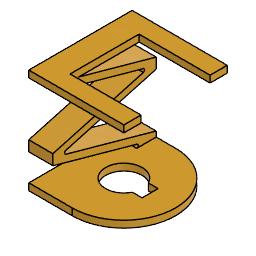
Keybord-Base (Autodesk Fusion 360 archive; units mm, degrees)
design "ボタン-スプリング"
Autodesk Fusion 360 part; units mm, degrees
note: some values were not read from the file. Set by a fixed rule: which face or edge a step refers to.
(part 1 of 3)
sketch "スケッチ1" plane through (0, 0, 0) normal (0, 0, 1) x (1, 0, 0)
  circle A0 centre (0, 0) radius 2.65
  line L0 (0, -7.5) -> (0, 7.5)
  line L1 (0, 7.5) -> (-6.3, 7.5)
  line L2 (-6.3, 7.5) -> (-6.3, -7.5)
  line L3 (-6.3, -7.5) -> (0, -7.5)
  line L4 (0, -7.5) -> (0, 7.5)
  arc A1 (0, -7.5) -> (0, 7.5) centre (0, 0) ccw
  line L5 (2.65, 0) -> (-2.65, 0)
  line L6 (3.8, 1.15) -> (1.5, 1.15)
  line L7 (1.5, 1.15) -> (1.5, -1.15)
  line L8 (1.5, -1.15) -> (3.8, -1.15)
  line L9 (3.8, -1.15) -> (3.8, 1.15)
  line L10 (3.8, 1.15) -> (1.5, -1.15) construction
  line L11 (1.5, 1.15) -> (3.8, -1.15) construction
  point P0 (2.65, 0)
  dimension "d1" = 5.3
  dimension "d2" = 15
  dimension "d5" = 6.3
  dimension "d6" = 15
  dimension "d31" = 2.3
  dimension "d32" = 2.3
  constraint coincident A0.centre A1.centre
  constraint midpoint L0 A0.centre
  constraint vertical L0
  constraint horizontal L1
  constraint vertical L2
  constraint horizontal L3
  constraint vertical L4
  constraint midpoint L5 A0.centre
  constraint coincident A0 L5.end
  constraint perpendicular L0 L5
  constraint horizontal L6
  constraint perpendicular L6 L7
  constraint parallel L6 L8
  constraint parallel L7 L9
  constraint coincident L10 P0
  constraint coincident L11 P0
  constraint coincident P0 L5.start
  measures "d1" diameter of A0
  measures "d2" diameter of A1
  measures "d5" distance of A0.centre L2
  measures "d6" distance of L1 L3
  measures "d31" distance of L7.end L8.end
  measures "d32" distance of L6.end L7.end
extrude "押し出し1" add sketch "スケッチ1" along normal blind 1 contours A0 L0 L4 A1 L6 L8 L9 | A0 L0 L1 L2 L3 L4
sketch "スケッチ2" plane through (-6.3, 0, 0) normal (-1, 0, 0) x (0, -1, 0)
  line L0 (-7.5, 0) -> (7.5, 0)
  line L1 (7.5, 0) -> (7.5, 1)
  line L2 (7.5, 1) -> (-7.5, 1)
  line L3 (-7.5, 1) -> (-7.5, 0)
  line L4 (-7.5, 1) -> (-7.5, 16) construction
  line L5 (7.5, 1) -> (7.5, 16) construction
  line L6 (-7.5, 1) -> (-7.5, 1.7604)
  line L7 (-6.5, 1) -> (-7.5, 1)
  line L8 (-7.5, 1) -> (-7.5, 1.7604)
  line L9 (-4.7298, 1.4909) -> (7.5, 4.8825)
  line L10 (-4.663, 1) -> (10.2045, 1) construction
  line L11 (-7.5, 1.7604) -> (5.6313, 5.4021)
  line L12 (5.6313, 5.8839) -> (-7.5, 9.5255)
  line L13 (-5.6313, 10.045) -> (7.5, 6.4034)
  line L14 (7.5, 6.4034) -> (7.5, 4.8825)
  line L15 (-5.6313, 10.5268) -> (7.5, 14.1685)
  line L16 (-7.5, 11.0463) -> (3.758, 14.1685)
  line L17 (-7.5, 11.0463) -> (-7.5, 9.5255)
  line L18 (7.5, 14.1685) -> (3.758, 14.1685)
  arc A0 (-4.7298, 1.4909) -> (-4.663, 1) centre (-4.663, 1.25) ccw
  arc A1 (5.6313, 5.4021) -> (5.6313, 5.8839) centre (5.5645, 5.643) ccw
  arc A2 (-5.6313, 10.5268) -> (-5.6313, 10.045) centre (-5.5645, 10.2859) ccw
  point P0 (6.5, 5.643)
  point P1 (-6.5, 10.2859)
  dimension "d7" = 15
  dimension "d8" = 15
  dimension "d9" = 15.5
  dimension "d15" = 15.5
  dimension "d16" = 1
  dimension "d17" = 1
  dimension "d18" = 15.5
  dimension "d19" = 15.5
  dimension "d20" = 1
  dimension "d21" = 1
  dimension "d22" = 15.5
  dimension "d23" = 15.5
  dimension "d24" = 1
  dimension "d25" = 1
  dimension "d26" = 0.25
  dimension "d27" = 0.25
  dimension "d28" = 0.25
  constraint coincident L2.end L3.start
  constraint perpendicular L2 L4
  constraint coincident L1.end L2.start
  constraint perpendicular L2 L5
  constraint coincident L4 L6.end
  constraint horizontal L7
  constraint vertical L8
  constraint coincident L2 L7.start
  constraint horizontal L10
  constraint coincident L5 L9.end
  constraint coincident L5 L13.end
  constraint coincident L4 L12.end
  constraint coincident L4 L16.start
  constraint coincident L5 L15.end
  constraint parallel L10 L18
  constraint coincident L7.start L9
  constraint coincident L7.start L10
  constraint tangent L9 A0
  constraint tangent L10 A0
  constraint coincident P0 L11
  constraint coincident P0 L12
  constraint tangent L11 A1
  constraint tangent L12 A1
  constraint coincident P1 L15
  constraint coincident P1 L13
  constraint tangent L15 A2
  constraint tangent L13 A2
  measures "d7" distance of L2.end L4.end
  measures "d8" distance of L1.end L5.end
  measures "d9" angle of L9 L10
  measures "d15" angle of L10 L11
  measures "d16" distance of L9 L11
  measures "d17" distance of L7.start L2.end
  measures "d18" angle of L10 L12
  measures "d19" angle of L10 L13
  measures "d20" distance of L12 L13
  measures "d21" distance of P0 L14
  measures "d22" angle of L10 L15
  measures "d23" angle of L10 L16
  measures "d24" distance of L15 L16
  measures "d25" distance of P1 L17
  measures "d26" radius of A0
  measures "d27" radius of A1
  measures "d28" radius of A2
extrude "押し出し2" add sketch "スケッチ2" against normal blind 3.5 contours L2 L6 L7 L8 L9 L11 L12 L13 L14 L15 L16 L17 L18 A0 A1 A2
sketch "スケッチ3" plane through (0, 0, 14.1685) normal (0, 0, 1) x (-1, 0, 0)
  line L0 (6.3, 3.758) -> (6.3, 7.5)
  line L1 (6.3, 7.5) -> (2.8, 7.5)
  line L2 (2.8, 7.5) -> (2.8, 3.758)
  line L3 (2.8, 3.758) -> (6.3, 3.758)
  line L4 (2.8, -4.663) -> (6.3, -4.663)
  line L5 (6.3, -4.663) -> (6.3, 7.5)
  line L6 (6.3, 7.5) -> (0, 7.5)
  arc A0 (0, 7.5) -> (0, -7.5) centre (0, 0) ccw
  line L7 (0, -7.5) -> (2.8, -7.5)
  line L8 (2.8, -7.5) -> (2.8, -4.663)
  line L9 (-3.8, -1.15) -> (-3.8, 1.15)
  line L10 (-3.8, 1.15) -> (-2.3875, 1.15)
  arc A1 (-2.3875, -1.15) -> (-2.3875, 1.15) centre (0, 0) ccw
  line L11 (-2.3875, -1.15) -> (-3.8, -1.15)
  line L12 (6.3, -7.5) -> (6.3, 3.758)
  line L13 (6.3, 3.758) -> (2.8, 3.758)
  line L14 (2.8, 3.758) -> (2.8, -7.5)
  line L15 (2.8, -7.5) -> (6.3, -7.5)
  line L16 (6.3, 5) -> (6.3, -5)
  line L17 (-7.5, 0) -> (-7.5, -7.5)
  line L18 (-7.5, -7.5) -> (6.3, -7.5)
  line L19 (6.3, -4.663) -> (6.3, -7.5)
  line L20 (6.3, -5) -> (-7.5, -5)
  line L21 (-20, 0) -> (-2.5, 0)
  line L22 (6.3, 5) -> (-7.5, 5)
  line L23 (-7.5, 0) -> (-7.5, 7.5)
  line L24 (6.3, 4.663) -> (6.3, 7.5)
  line L25 (-7.5, 7.5) -> (6.3, 7.5)
  point P0 (6.3, 0)
  dimension "d38" = 5
  constraint midpoint L16 P0
  constraint coincident L12 P0
  constraint coincident L12 L16.end
  constraint midpoint A0 L17.start
  constraint tangent A0 L17
  constraint perpendicular L7 L17
  constraint coincident L12.start L15.end
  constraint perpendicular L12 L18
  constraint coincident L4.end L5.start
  constraint coincident L17 L20.end
  constraint perpendicular L17 L20
  constraint symmetric L17.start L21 L23.start
  constraint symmetric L17.end L21 L23.end
  constraint symmetric L12.start L21 L0.end
  constraint symmetric L4.end L21 L24.start
  constraint symmetric L16.end L21 L16.start
  constraint symmetric L20.end L21 L22.end
  measures "d38" distance of A0.centre L20
extrude "押し出し3" add sketch "スケッチ3" along normal blind 1 contours L0 L2 L3 L5 L13 L16 L22 L24 | L3 L4 L5 L12 L13 L14 L16 | L4 L8 L12 L14 L16 L19 L20 | L0 L1 L2 L5 L6 L22 L24 L25 | L2 L6 A0 L22 L25 | L8 L12 L14 L15 L18 L19 L20 | A0 L22 L23 L25 | A0 L7 L8 L14 L18 L20 | A0 L17 L18 L20
equation "d5 = d1 + 1 mm"
equation "d6 = d2"
equation "d8 = d7"
equation "d15 = d9"
equation "d17 = d16"
equation "d18 = d9"
equation "d19 = d9"
equation "d20 = d16"
equation "d21 = d16"
equation "d22 = d9"
equation "d23 = d9"
equation "d24 = d16"
equation "d25 = d16"
equation "d31 = d32"

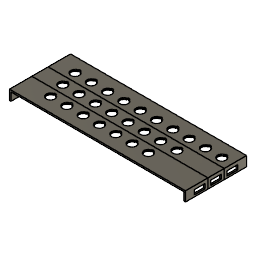
design "Keybord-Base-top"
Autodesk Fusion 360 part; units mm, degrees
sketch "スケッチ1" plane through (0, 0, 0) normal (0, 0, 1) x (1, 0, 0)
  circle A0 centre (0, 0) radius 4.75
  line L0 (1.25, 3.5) -> (-1.25, 3.5)
  line L1 (-1.25, 3.5) -> (-1.25, 6)
  line L2 (-1.25, 6) -> (1.25, 6)
  line L3 (1.25, 6) -> (1.25, 3.5)
  line L4 (1.25, 3.5) -> (-1.25, 6) construction
  line L5 (-1.25, 3.5) -> (1.25, 6) construction
  line L6 (0, -6.2565) -> (0, 6.2565)
  line L7 (-5.8047, 0) -> (5.8047, 0)
  circle A1 centre (20, 0) radius 4.75
  line L8 (18.75, 3.5) -> (21.25, 6) construction
  line L9 (14.1953, 0) -> (25.8047, 0)
  line L10 (20, -6.2565) -> (20, 6.2565)
  line L11 (18.75, 6) -> (21.25, 6)
  line L12 (18.75, 3.5) -> (18.75, 6)
  line L13 (21.25, 3.5) -> (18.75, 6) construction
  line L14 (21.25, 6) -> (21.25, 3.5)
  line L15 (21.25, 3.5) -> (18.75, 3.5)
  circle A2 centre (40, 0) radius 4.75
  line L16 (38.75, 3.5) -> (41.25, 6) construction
  line L17 (34.1953, 0) -> (45.8047, 0)
  line L18 (40, -6.2565) -> (40, 6.2565)
  line L19 (38.75, 6) -> (41.25, 6)
  line L20 (38.75, 3.5) -> (38.75, 6)
  line L21 (41.25, 3.5) -> (38.75, 6) construction
  line L22 (41.25, 6) -> (41.25, 3.5)
  line L23 (41.25, 3.5) -> (38.75, 3.5)
  circle A3 centre (60, 0) radius 4.75
  line L24 (58.75, 3.5) -> (61.25, 6) construction
  line L25 (54.1953, 0) -> (65.8047, 0)
  line L26 (60, -6.2565) -> (60, 6.2565)
  line L27 (58.75, 6) -> (61.25, 6)
  line L28 (58.75, 3.5) -> (58.75, 6)
  line L29 (61.25, 3.5) -> (58.75, 6) construction
  line L30 (61.25, 6) -> (61.25, 3.5)
  line L31 (61.25, 3.5) -> (58.75, 3.5)
  line L32 (-21.25, 3.5) -> (-18.75, 6) construction
  line L33 (-18.75, 6) -> (-18.75, 3.5)
  line L34 (-25.8047, 0) -> (-14.1953, 0)
  line L35 (-21.25, 3.5) -> (-21.25, 6)
  line L36 (-20, -6.2565) -> (-20, 6.2565)
  line L37 (-21.25, 6) -> (-18.75, 6)
  circle A4 centre (-20, 0) radius 4.75
  line L38 (-18.75, 3.5) -> (-21.25, 6) construction
  line L39 (-18.75, 3.5) -> (-21.25, 3.5)
  line L40 (-41.25, 3.5) -> (-38.75, 6) construction
  line L41 (-38.75, 6) -> (-38.75, 3.5)
  line L42 (-45.8047, 0) -> (-34.1953, 0)
  line L43 (-41.25, 3.5) -> (-41.25, 6)
  line L44 (-40, -6.2565) -> (-40, 6.2565)
  line L45 (-41.25, 6) -> (-38.75, 6)
  circle A5 centre (-40, 0) radius 4.75
  line L46 (-38.75, 3.5) -> (-41.25, 6) construction
  line L47 (-38.75, 3.5) -> (-41.25, 3.5)
  line L48 (-61.25, 3.5) -> (-58.75, 6) construction
  line L49 (-58.75, 6) -> (-58.75, 3.5)
  line L50 (-65.8047, 0) -> (-54.1953, 0)
  line L51 (-61.25, 3.5) -> (-61.25, 6)
  line L52 (-60, -6.2565) -> (-60, 6.2565)
  line L53 (-61.25, 6) -> (-58.75, 6)
  circle A6 centre (-60, 0) radius 4.75
  line L54 (-58.75, 3.5) -> (-61.25, 6) construction
  line L55 (-58.75, 3.5) -> (-61.25, 3.5)
  line L56 (-81.25, 3.5) -> (-78.75, 6) construction
  line L57 (-78.75, 6) -> (-78.75, 3.5)
  line L58 (-85.8047, 0) -> (-74.1953, 0)
  line L59 (-81.25, 3.5) -> (-81.25, 6)
  line L60 (-80, -6.2565) -> (-80, 6.2565)
  line L61 (-81.25, 6) -> (-78.75, 6)
  circle A7 centre (-80, 0) radius 4.75
  line L62 (-78.75, 3.5) -> (-81.25, 6) construction
  line L63 (-78.75, 3.5) -> (-81.25, 3.5)
  line L64 (-3.75, 23.5) -> (-6.25, 23.5)
  line L65 (-3.75, 23.5) -> (-6.25, 26) construction
  line L66 (-10.8047, 20) -> (0.8047, 20)
  line L67 (-6.25, 23.5) -> (-6.25, 26)
  line L68 (-6.25, 23.5) -> (-3.75, 26) construction
  line L69 (-6.25, 26) -> (-3.75, 26)
  line L70 (-5, 13.7435) -> (-5, 26.2565)
  line L71 (-3.75, 26) -> (-3.75, 23.5)
  circle A8 centre (-5, 20) radius 4.75
  line L72 (16.25, 23.5) -> (13.75, 23.5)
  line L73 (13.75, 23.5) -> (13.75, 26)
  line L74 (16.25, 23.5) -> (13.75, 26) construction
  circle A9 centre (15, 20) radius 4.75
  line L75 (13.75, 23.5) -> (16.25, 26) construction
  line L76 (9.1953, 20) -> (20.8047, 20)
  line L77 (15, 13.7435) -> (15, 26.2565)
  line L78 (13.75, 26) -> (16.25, 26)
  line L79 (16.25, 26) -> (16.25, 23.5)
  line L80 (36.25, 23.5) -> (33.75, 23.5)
  line L81 (33.75, 23.5) -> (33.75, 26)
  line L82 (36.25, 23.5) -> (33.75, 26) construction
  circle A10 centre (35, 20) radius 4.75
  line L83 (33.75, 23.5) -> (36.25, 26) construction
  line L84 (29.1953, 20) -> (40.8047, 20)
  line L85 (35, 13.7435) -> (35, 26.2565)
  line L86 (33.75, 26) -> (36.25, 26)
  line L87 (36.25, 26) -> (36.25, 23.5)
  line L88 (56.25, 23.5) -> (53.75, 23.5)
  line L89 (53.75, 23.5) -> (53.75, 26)
  line L90 (56.25, 23.5) -> (53.75, 26) construction
  circle A11 centre (55, 20) radius 4.75
  line L91 (53.75, 23.5) -> (56.25, 26) construction
  line L92 (49.1953, 20) -> (60.8047, 20)
  line L93 (55, 13.7435) -> (55, 26.2565)
  line L94 (53.75, 26) -> (56.25, 26)
  line L95 (56.25, 26) -> (56.25, 23.5)
  line L96 (76.25, 23.5) -> (73.75, 23.5)
  line L97 (73.75, 23.5) -> (73.75, 26)
  line L98 (76.25, 23.5) -> (73.75, 26) construction
  circle A12 centre (75, 20) radius 4.75
  line L99 (73.75, 23.5) -> (76.25, 26) construction
  line L100 (69.1953, 20) -> (80.8047, 20)
  line L101 (75, 13.7435) -> (75, 26.2565)
  line L102 (73.75, 26) -> (76.25, 26)
  line L103 (76.25, 26) -> (76.25, 23.5)
  line L104 (96.25, 23.5) -> (93.75, 23.5)
  line L105 (93.75, 23.5) -> (93.75, 26)
  line L106 (96.25, 23.5) -> (93.75, 26) construction
  circle A13 centre (95, 20) radius 4.75
  line L107 (93.75, 23.5) -> (96.25, 26) construction
  line L108 (89.1953, 20) -> (100.8047, 20)
  line L109 (95, 13.7435) -> (95, 26.2565)
  line L110 (93.75, 26) -> (96.25, 26)
  line L111 (96.25, 26) -> (96.25, 23.5)
  line L112 (-23.75, 26) -> (-23.75, 23.5)
  line L113 (-23.75, 23.5) -> (-26.25, 23.5)
  circle A14 centre (-25, 20) radius 4.75
  line L114 (-23.75, 23.5) -> (-26.25, 26) construction
  line L115 (-30.8047, 20) -> (-19.1953, 20)
  line L116 (-25, 13.7435) -> (-25, 26.2565)
  line L117 (-26.25, 23.5) -> (-26.25, 26)
  line L118 (-26.25, 26) -> (-23.75, 26)
  line L119 (-26.25, 23.5) -> (-23.75, 26) construction
  line L120 (-43.75, 26) -> (-43.75, 23.5)
  line L121 (-43.75, 23.5) -> (-46.25, 23.5)
  circle A15 centre (-45, 20) radius 4.75
  line L122 (-43.75, 23.5) -> (-46.25, 26) construction
  line L123 (-50.8047, 20) -> (-39.1953, 20)
  line L124 (-45, 13.7435) -> (-45, 26.2565)
  line L125 (-46.25, 23.5) -> (-46.25, 26)
  line L126 (-46.25, 26) -> (-43.75, 26)
  line L127 (-46.25, 23.5) -> (-43.75, 26) construction
  line L128 (-63.75, 26) -> (-63.75, 23.5)
  line L129 (-63.75, 23.5) -> (-66.25, 23.5)
  circle A16 centre (-65, 20) radius 4.75
  line L130 (-63.75, 23.5) -> (-66.25, 26) construction
  line L131 (-70.8047, 20) -> (-59.1953, 20)
  line L132 (-65, 13.7435) -> (-65, 26.2565)
  line L133 (-66.25, 23.5) -> (-66.25, 26)
  line L134 (-66.25, 26) -> (-63.75, 26)
  line L135 (-66.25, 23.5) -> (-63.75, 26) construction
  line L136 (-83.75, 26) -> (-83.75, 23.5)
  line L137 (-83.75, 23.5) -> (-86.25, 23.5)
  circle A17 centre (-85, 20) radius 4.75
  line L138 (-83.75, 23.5) -> (-86.25, 26) construction
  line L139 (-90.8047, 20) -> (-79.1953, 20)
  line L140 (-85, 13.7435) -> (-85, 26.2565)
  line L141 (-86.25, 23.5) -> (-86.25, 26)
  line L142 (-86.25, 26) -> (-83.75, 26)
  line L143 (-86.25, 23.5) -> (-83.75, 26) construction
  circle A18 centre (5, -20) radius 4.75
  line L144 (3.75, -14) -> (6.25, -14)
  line L145 (6.25, -14) -> (6.25, -16.5)
  line L146 (3.75, -16.5) -> (3.75, -14)
  line L147 (6.25, -16.5) -> (3.75, -16.5)
  line L148 (6.25, -16.5) -> (3.75, -14) construction
  line L149 (3.75, -16.5) -> (6.25, -14) construction
  line L150 (-0.8294, -20) -> (10.7799, -20)
  line L151 (5, -26.3014) -> (5, -13.7884)
  line L152 (26.25, -16.5) -> (23.75, -16.5)
  circle A19 centre (25, -20) radius 4.75
  line L153 (23.75, -14) -> (26.25, -14)
  line L154 (26.25, -16.5) -> (23.75, -14) construction
  line L155 (25, -26.3014) -> (25, -13.7884)
  line L156 (23.75, -16.5) -> (23.75, -14)
  line L157 (23.75, -16.5) -> (26.25, -14) construction
  line L158 (19.1706, -20) -> (30.7799, -20)
  line L159 (26.25, -14) -> (26.25, -16.5)
  line L160 (46.25, -16.5) -> (43.75, -16.5)
  circle A20 centre (45, -20) radius 4.75
  line L161 (43.75, -14) -> (46.25, -14)
  line L162 (46.25, -16.5) -> (43.75, -14) construction
  line L163 (45, -26.3014) -> (45, -13.7884)
  line L164 (43.75, -16.5) -> (43.75, -14)
  line L165 (43.75, -16.5) -> (46.25, -14) construction
  line L166 (39.1706, -20) -> (50.7799, -20)
  line L167 (46.25, -14) -> (46.25, -16.5)
  line L168 (-16.25, -16.5) -> (-16.25, -14)
  line L169 (-13.75, -16.5) -> (-16.25, -14) construction
  circle A21 centre (-15, -20) radius 4.75
  line L170 (-16.25, -16.5) -> (-13.75, -14) construction
  line L171 (-15, -26.3014) -> (-15, -13.7884)
  line L172 (-16.25, -14) -> (-13.75, -14)
  line L173 (-13.75, -16.5) -> (-16.25, -16.5)
  line L174 (-13.75, -14) -> (-13.75, -16.5)
  line L175 (-20.8294, -20) -> (-9.2201, -20)
  line L176 (-36.25, -16.5) -> (-36.25, -14)
  line L177 (-33.75, -16.5) -> (-36.25, -14) construction
  circle A22 centre (-35, -20) radius 4.75
  line L178 (-36.25, -16.5) -> (-33.75, -14) construction
  line L179 (-35, -26.3014) -> (-35, -13.7884)
  line L180 (-36.25, -14) -> (-33.75, -14)
  line L181 (-33.75, -16.5) -> (-36.25, -16.5)
  line L182 (-33.75, -14) -> (-33.75, -16.5)
  line L183 (-40.8294, -20) -> (-29.2201, -20)
  line L184 (-56.25, -16.5) -> (-56.25, -14)
  line L185 (-53.75, -16.5) -> (-56.25, -14) construction
  circle A23 centre (-55, -20) radius 4.75
  line L186 (-56.25, -16.5) -> (-53.75, -14) construction
  line L187 (-55, -26.3014) -> (-55, -13.7884)
  line L188 (-56.25, -14) -> (-53.75, -14)
  line L189 (-53.75, -16.5) -> (-56.25, -16.5)
  line L190 (-53.75, -14) -> (-53.75, -16.5)
  line L191 (-60.8294, -20) -> (-49.2201, -20)
  line L192 (-76.25, -16.5) -> (-76.25, -14)
  line L193 (-73.75, -16.5) -> (-76.25, -14) construction
  circle A24 centre (-75, -20) radius 4.75
  line L194 (-76.25, -16.5) -> (-73.75, -14) construction
  line L195 (-75, -26.3014) -> (-75, -13.7884)
  line L196 (-76.25, -14) -> (-73.75, -14)
  line L197 (-73.75, -16.5) -> (-76.25, -16.5)
  line L198 (-73.75, -14) -> (-73.75, -16.5)
  line L199 (-80.8294, -20) -> (-69.2201, -20)
  line L200 (108, 37.5) -> (-108, 37.5)
  line L201 (-108, 37.5) -> (-108, -37.5)
  line L202 (-108, -37.5) -> (108, -37.5)
  line L203 (108, -37.5) -> (108, 37.5)
  line L204 (108, 37.5) -> (-108, -37.5) construction
  line L205 (-108, 37.5) -> (108, -37.5) construction
  point P0 (0, 4.75)
  point P1 (20, 0)
  point P2 (20, 0)
  point P3 (20, 4.75)
  point P4 (20, 0)
  point P5 (20, 0)
  point P6 (40, 0)
  point P7 (40, 0)
  point P8 (40, 4.75)
  point P9 (40, 0)
  point P10 (40, 0)
  point P11 (60, 0)
  point P12 (60, 0)
  point P13 (60, 4.75)
  point P14 (60, 0)
  point P15 (60, 0)
  point P16 (-20, 0)
  point P17 (-20, 0)
  point P18 (-20, 0)
  point P19 (-20, 0)
  point P20 (-20, 4.75)
  point P21 (-40, 0)
  point P22 (-40, 0)
  point P23 (-40, 0)
  point P24 (-40, 0)
  point P25 (-40, 4.75)
  point P26 (-60, 0)
  point P27 (-60, 0)
  point P28 (-60, 0)
  point P29 (-60, 0)
  point P30 (-60, 4.75)
  point P31 (-80, 0)
  point P32 (-80, 0)
  point P33 (-80, 0)
  point P34 (-80, 0)
  point P35 (-80, 4.75)
  point P36 (25.8047, 17)
  point P37 (-5, 20)
  point P38 (14.1953, 17)
  point P39 (-5, 24.75)
  point P40 (-5, 20)
  point P41 (-5, 20)
  point P42 (-5, 20)
  point P43 (15, 24.75)
  point P44 (15, 20)
  point P45 (15, 20)
  point P46 (15, 20)
  point P47 (15, 20)
  point P48 (35, 24.75)
  point P49 (35, 20)
  point P50 (35, 20)
  point P51 (35, 20)
  point P52 (35, 20)
  point P53 (55, 24.75)
  point P54 (55, 20)
  point P55 (55, 20)
  point P56 (55, 20)
  point P57 (55, 20)
  point P58 (75, 24.75)
  point P59 (75, 20)
  point P60 (75, 20)
  point P61 (75, 20)
  point P62 (75, 20)
  point P63 (95, 24.75)
  point P64 (95, 20)
  point P65 (95, 20)
  point P66 (95, 20)
  point P67 (95, 20)
  point P68 (-25, 20)
  point P69 (-25, 20)
  point P70 (-25, 24.75)
  point P71 (-25, 20)
  point P72 (-25, 20)
  point P73 (-45, 20)
  point P74 (-45, 20)
  point P75 (-45, 24.75)
  point P76 (-45, 20)
  point P77 (-45, 20)
  point P78 (-65, 20)
  point P79 (-65, 20)
  point P80 (-65, 24.75)
  point P81 (-65, 20)
  point P82 (-65, 20)
  point P83 (-85, 20)
  point P84 (-85, 20)
  point P85 (-85, 24.75)
  point P86 (-85, 20)
  point P87 (-85, 20)
  point P88 (5, -15.25)
  point P89 (25, -15.25)
  point P90 (45, -15.25)
  point P91 (-15, -15.25)
  point P92 (-35, -15.25)
  point P93 (-55, -15.25)
  point P94 (-75, -15.25)
  dimension "d1" = 9.5
  dimension "d2" = 2.5
  dimension "d3" = 2.5
  dimension "d10" = 20
  dimension "d11" = 0
  dimension "d14" = -20
  dimension "d15" = 0
  dimension "d24" = 9.5
  dimension "d25" = 2.5
  dimension "d26" = 2.5
  dimension "d29" = 5
  dimension "d30" = 20
  dimension "d33" = 20
  dimension "d34" = 0
  dimension "d37" = -20
  dimension "d38" = 0
  dimension "d39" = 9.5
  dimension "d40" = 2.5
  dimension "d41" = 2.5
  dimension "d42" = 20
  dimension "d43" = 5
  dimension "d46" = 20
  dimension "d47" = 0
  dimension "d50" = -20
  dimension "d51" = 0
  dimension "d52" = 216
  dimension "d53" = 75
  constraint coincident A0.centre origin
  constraint horizontal L0
  constraint perpendicular L0 L1
  constraint parallel L0 L2
  constraint parallel L1 L3
  constraint coincident L4 P0
  constraint coincident L5 P0
  constraint coincident A0 P0
  constraint midpoint L6 A0.centre
  constraint perpendicular L2 L6
  constraint coincident P0 L6
  constraint midpoint L7 A0.centre
  constraint perpendicular L6 L7
  constraint coincident P42 P41
  constraint horizontal L64
  constraint perpendicular L64 L67
  constraint parallel L64 L69
  constraint parallel L67 L71
  constraint coincident P39 L65
  constraint coincident P39 L68
  constraint coincident P39 A8
  constraint midpoint P42 L70
  constraint perpendicular L69 L70
  constraint coincident P39 L70
  constraint midpoint P42 L66
  constraint perpendicular L66 L70
  constraint horizontal L147
  constraint perpendicular L146 L147
  constraint parallel L144 L147
  constraint parallel L145 L146
  constraint perpendicular L144 L151
  constraint perpendicular L150 L151
  constraint midpoint L148 P88
  constraint coincident A18 P88
  constraint coincident A18.centre L151
  constraint coincident A18.centre L150
  constraint coincident L151 P88
  constraint horizontal L200
  constraint perpendicular L200 L201
  constraint parallel L200 L202
  constraint parallel L201 L203
  constraint coincident L204 A0.centre
  constraint coincident L205 A0.centre
  measures "d1" diameter of A0
  measures "d2" distance of L1.end L2.end
  measures "d3" distance of L0.end L1.end
  measures "d24" diameter of A8
  measures "d25" distance of L65.end L68.end
  measures "d26" distance of L65.end L64.end
  measures "d29" horizontal distance of A0.centre P42
  measures "d30" vertical distance of A0.centre P42
  measures "d39" diameter of A18
  measures "d40" distance of L144.start L144.end
  measures "d41" distance of L144.start L146.start
  measures "d42" vertical distance of A0.centre A18.centre
  measures "d43" horizontal distance of A0.centre A18.centre
  measures "d52" distance of L200.start L200.end
  measures "d53" distance of L200.start L202.end
extrude "押し出し1" add sketch "スケッチ1" along normal blind 2 makes body 1
sketch "スケッチ2" plane through (0, 0, 0) normal (0, 0, -1) x (1, 0, 0)
  arc A0 (-63.75, -24.5826) -> (-66.25, -24.5826) centre (-65, -20) ccw
  line L0 (-63.75, -24.5826) -> (-63.75, -26)
  line L1 (-63.75, -26) -> (-66.25, -26)
  line L2 (-66.25, -26) -> (-66.25, -24.5826)
  line L3 (-21.25, -6) -> (-21.25, -4.5826)
  arc A1 (-18.75, -4.5826) -> (-21.25, -4.5826) centre (-20, 0) ccw
  line L4 (-18.75, -4.5826) -> (-18.75, -6)
  line L5 (-18.75, -6) -> (-21.25, -6)
  line L6 (-61.25, -6) -> (-61.25, -4.5826)
  arc A2 (-58.75, -4.5826) -> (-61.25, -4.5826) centre (-60, 0) ccw
  line L7 (-58.75, -4.5826) -> (-58.75, -6)
  line L8 (-58.75, -6) -> (-61.25, -6)
  line L9 (-81.25, -6) -> (-81.25, -4.5826)
  arc A3 (-78.75, -4.5826) -> (-81.25, -4.5826) centre (-80, 0) ccw
  line L10 (-78.75, -4.5826) -> (-78.75, -6)
  line L11 (-78.75, -6) -> (-81.25, -6)
  line L12 (3.75, 14) -> (3.75, 15.4174)
  arc A4 (6.25, 15.4174) -> (3.75, 15.4174) centre (5, 20) ccw
  line L13 (6.25, 15.4174) -> (6.25, 14)
  line L14 (6.25, 14) -> (3.75, 14)
  arc A5 (-43.75, -24.5826) -> (-46.25, -24.5826) centre (-45, -20) ccw
  line L15 (-43.75, -24.5826) -> (-43.75, -26)
  line L16 (-43.75, -26) -> (-46.25, -26)
  line L17 (-46.25, -26) -> (-46.25, -24.5826)
  arc A6 (-13.75, 15.4174) -> (-16.25, 15.4174) centre (-15, 20) ccw
  line L18 (-13.75, 15.4174) -> (-13.75, 14)
  line L19 (-13.75, 14) -> (-16.25, 14)
  line L20 (-16.25, 14) -> (-16.25, 15.4174)
  arc A7 (26.25, 15.4174) -> (23.75, 15.4174) centre (25, 20) ccw
  line L21 (26.25, 15.4174) -> (26.25, 14)
  line L22 (26.25, 14) -> (23.75, 14)
  line L23 (23.75, 14) -> (23.75, 15.4174)
  arc A8 (-83.75, -24.5826) -> (-86.25, -24.5826) centre (-85, -20) ccw
  line L24 (-83.75, -24.5826) -> (-83.75, -26)
  line L25 (-83.75, -26) -> (-86.25, -26)
  line L26 (-86.25, -26) -> (-86.25, -24.5826)
  line L27 (-41.25, -6) -> (-41.25, -4.5826)
  arc A9 (-38.75, -4.5826) -> (-41.25, -4.5826) centre (-40, 0) ccw
  line L28 (-38.75, -4.5826) -> (-38.75, -6)
  line L29 (-38.75, -6) -> (-41.25, -6)
  arc A10 (-33.75, 15.4174) -> (-36.25, 15.4174) centre (-35, 20) ccw
  line L30 (-33.75, 15.4174) -> (-33.75, 14)
  line L31 (-33.75, 14) -> (-36.25, 14)
  line L32 (-36.25, 14) -> (-36.25, 15.4174)
  arc A11 (96.25, -24.5826) -> (93.75, -24.5826) centre (95, -20) ccw
  line L33 (96.25, -24.5826) -> (96.25, -26)
  line L34 (96.25, -26) -> (93.75, -26)
  line L35 (93.75, -26) -> (93.75, -24.5826)
  line L36 (-6.25, -26) -> (-6.25, -24.5826)
  arc A12 (-3.75, -24.5826) -> (-6.25, -24.5826) centre (-5, -20) ccw
  line L37 (-3.75, -24.5826) -> (-3.75, -26)
  line L38 (-3.75, -26) -> (-6.25, -26)
  arc A13 (-53.75, 15.4174) -> (-56.25, 15.4174) centre (-55, 20) ccw
  line L39 (-53.75, 15.4174) -> (-53.75, 14)
  line L40 (-53.75, 14) -> (-56.25, 14)
  line L41 (-56.25, 14) -> (-56.25, 15.4174)
  arc A14 (76.25, -24.5826) -> (73.75, -24.5826) centre (75, -20) ccw
  line L42 (76.25, -24.5826) -> (76.25, -26)
  line L43 (76.25, -26) -> (73.75, -26)
  line L44 (73.75, -26) -> (73.75, -24.5826)
  arc A15 (46.25, 15.4174) -> (43.75, 15.4174) centre (45, 20) ccw
  line L45 (46.25, 15.4174) -> (46.25, 14)
  line L46 (46.25, 14) -> (43.75, 14)
  line L47 (43.75, 14) -> (43.75, 15.4174)
  arc A16 (36.25, -24.5826) -> (33.75, -24.5826) centre (35, -20) ccw
  line L48 (36.25, -24.5826) -> (36.25, -26)
  line L49 (36.25, -26) -> (33.75, -26)
  line L50 (33.75, -26) -> (33.75, -24.5826)
  arc A17 (56.25, -24.5826) -> (53.75, -24.5826) centre (55, -20) ccw
  line L51 (56.25, -24.5826) -> (56.25, -26)
  line L52 (56.25, -26) -> (53.75, -26)
  line L53 (53.75, -26) -> (53.75, -24.5826)
  arc A18 (-73.75, 15.4174) -> (-76.25, 15.4174) centre (-75, 20) ccw
  line L54 (-73.75, 15.4174) -> (-73.75, 14)
  line L55 (-73.75, 14) -> (-76.25, 14)
  line L56 (-76.25, 14) -> (-76.25, 15.4174)
  arc A19 (1.25, -4.5826) -> (-1.25, -4.5826) centre (0, 0) ccw
  line L57 (1.25, -4.5826) -> (1.25, -6)
  line L58 (1.25, -6) -> (-1.25, -6)
  line L59 (-1.25, -6) -> (-1.25, -4.5826)
  arc A20 (16.25, -24.5826) -> (13.75, -24.5826) centre (15, -20) ccw
  line L60 (16.25, -24.5826) -> (16.25, -26)
  line L61 (16.25, -26) -> (13.75, -26)
  line L62 (13.75, -26) -> (13.75, -24.5826)
  arc A21 (41.25, -4.5826) -> (38.75, -4.5826) centre (40, 0) ccw
  line L63 (41.25, -4.5826) -> (41.25, -6)
  line L64 (41.25, -6) -> (38.75, -6)
  line L65 (38.75, -6) -> (38.75, -4.5826)
  arc A22 (-23.75, -24.5826) -> (-26.25, -24.5826) centre (-25, -20) ccw
  line L66 (-23.75, -24.5826) -> (-23.75, -26)
  line L67 (-23.75, -26) -> (-26.25, -26)
  line L68 (-26.25, -26) -> (-26.25, -24.5826)
  arc A23 (21.25, -4.5826) -> (18.75, -4.5826) centre (20, 0) ccw
  line L69 (21.25, -4.5826) -> (21.25, -6)
  line L70 (21.25, -6) -> (18.75, -6)
  line L71 (18.75, -6) -> (18.75, -4.5826)
  arc A24 (61.25, -4.5826) -> (58.75, -4.5826) centre (60, 0) ccw
  line L72 (61.25, -4.5826) -> (61.25, -6)
  line L73 (61.25, -6) -> (58.75, -6)
  line L74 (58.75, -6) -> (58.75, -4.5826)
  line L75 (108, -37.5) -> (108, 37.5)
  line L76 (108, 37.5) -> (-108, 37.5)
  line L77 (-108, 37.5) -> (-108, -37.5)
  line L78 (-108, -37.5) -> (108, -37.5)
  line L79 (108, -37.5) -> (106, -37.5)
  line L80 (106, -37.5) -> (106, 37.525)
  line L81 (106, 37.525) -> (108, 37.525)
  line L82 (108, 37.525) -> (108, -37.5)
  line L83 (-108, -37.5) -> (-106, -37.5)
  line L84 (-106, -37.5) -> (-106, 37.525)
  line L85 (-106, 37.525) -> (-108, 37.525)
  line L86 (-108, 37.525) -> (-108, -37.5)
  dimension "d56" = 2
  dimension "d57" = 2
  constraint horizontal L79
  constraint vertical L80
  constraint horizontal L81
  constraint vertical L82
  constraint coincident L75.start L78.end
  constraint horizontal L83
  constraint vertical L84
  constraint horizontal L85
  constraint vertical L86
  constraint coincident L77.end L78.start
  measures "d56" distance of L75.start L79.end
  measures "d57" distance of L77.end L83.end
extrude "押し出し2" add sketch "スケッチ2" along normal blind 10 contours L75 L76 L78 L79 L80 L82 | L76 L80 L81 L82 | L76 L77 L78 L83 L84 L86 bodies 1
sketch "スケッチ3" plane through (108, 0, 0) normal (1, 0, 0) x (0, 1, 0)
  line L0 (37.5, -10) -> (37.5, 2)
  line L1 (37.5, 2) -> (-37.5, 2)
  line L2 (-37.5, 2) -> (-37.5, 0)
  line L3 (6.5, -7.75) -> (-6.5, -7.75)
  line L4 (-6.5, -7.75) -> (-6.5, -2.25)
  line L5 (-6.5, -2.25) -> (6.5, -2.25)
  line L6 (6.5, -2.25) -> (6.5, -7.75)
  line L7 (6.5, -7.75) -> (-6.5, -2.25) construction
  line L8 (-6.5, -7.75) -> (6.5, -2.25) construction
  line L9 (15.25, 0) -> (24.5826, 0)
  line L10 (24.5826, 0) -> (24.5826, 2)
  line L11 (15.25, 2) -> (24.5826, 2)
  line L12 (24.5826, 2) -> (24.5826, 0)
  line L13 (37.5, 0) -> (-37.5, 0)
  line L14 (-26.5, -2.25) -> (-13.5, -2.25)
  line L15 (-13.5, -2.25) -> (-13.5, -7.75)
  line L16 (-26.5, -7.75) -> (-26.5, -2.25)
  line L17 (-13.5, -7.75) -> (-26.5, -7.75)
  line L18 (-13.5, -7.75) -> (-26.5, -2.25) construction
  line L19 (-26.5, -7.75) -> (-13.5, -2.25) construction
  line L20 (13.5, -2.25) -> (26.5, -2.25)
  line L21 (26.5, -2.25) -> (26.5, -7.75)
  line L22 (13.5, -7.75) -> (13.5, -2.25)
  line L23 (26.5, -7.75) -> (13.5, -7.75)
  line L24 (26.5, -7.75) -> (13.5, -2.25) construction
  line L25 (13.5, -7.75) -> (26.5, -2.25) construction
  line L26 (-37.5, 0) -> (-37.525, 0)
  line L27 (-37.525, 0) -> (-37.525, -10)
  line L28 (-37.525, -10) -> (37.5, -10)
  line L29 (-4.75, 0) -> (4.5826, 0)
  line L30 (4.5826, 0) -> (4.5826, 2)
  line L31 (-4.75, 2) -> (4.5826, 2)
  line L32 (4.5826, 2) -> (4.5826, 0)
  line L33 (-24.75, 0) -> (-15.4174, 0)
  line L34 (-15.4174, 0) -> (-15.4174, 2)
  line L35 (-24.75, 2) -> (-15.4174, 2)
  line L36 (-15.4174, 2) -> (-15.4174, 0)
  point P0 (0, -5)
  point P1 (-20, -5)
  point P2 (20, -5)
  dimension "d60" = 5.5
  dimension "d61" = 13
  dimension "d62" = 5
  dimension "d65" = 20
  dimension "d66" = 0
  constraint horizontal L3
  constraint perpendicular L3 L4
  constraint parallel L3 L5
  constraint parallel L4 L6
  constraint coincident L7 P0
  constraint coincident L8 P0
  constraint vertical origin P0
  measures "d60" distance of L3.end L4.end
  measures "d61" distance of L4.end L5.end
  measures "d62" distance of P0 L13
extrude "押し出し3" cut sketch "スケッチ3" against normal up to surface (216 mm away) contours L3 L4 L5 L6 | L14 L15 L16 L17 | L20 L21 L22 L23 bodies 1
fillet "フィレット1" radius 0.5 25 faces at (-79.1869, -4.6799, 1.3333) (-83.7315, 15.4225, 1.3333) (-78.6002, -23.0986, 0.6667) (-57.5441, -24.0112, 0.6667) (-63.7363, 2.9331, 1.3333) (-66.4918, 15.4904, 1.3333) (-46.4918, 15.4904, 1.3333) (-42.1211, 4.2501, 1.3333) (-37.5441, -24.0112, 0.6667) (-19.4343, -21.7027, 1.3333) (-15.42, -1.2592, 0.6667) (-27.1211, 24.2501, 1.3333) (-9.4274, 21.7205, 1.3333) (-4.7154, -0.5727, 1.3333) (0.2622, -20.3403, 1.3333) (21.3998, -23.0986, 0.6667) (24.58, -1.2592, 0.6667) (10.2622, 19.6597, 1.3333) (33.5082, 15.4904, 0.6667) (53.5082, 15.4904, 1.3333) (76.2685, 15.4225, 1.3333) (96.2685, 15.4225, 1.3333) (37.8789, 4.2501, 1.3333) (64.1266, 2.3523, 0.6667) (42.4559, -24.0112, 0.6667) on bodies 1
ref_plane "作業平面1" through (0, 10, 0) normal (0, 1, 0) x (0, 0, 1)
ref_plane "作業平面2" through (0, -10, 0) normal (0, 1, 0) x (0, 0, 1)
split "分割1" by plane through (0, 10, 0) normal (0, 1, 0) and through (0, -10, 0) normal (0, 1, 0) bodies 1 makes body 2 at (-102.0662, 22.7445, 2) makes body 3 at (93.7499, -0.0151, 2)
copy_body "ボディ -> コンポーネント1" bodies 1 removing the originals makes body 4 in component "下段"
copy_body "ボディ -> コンポーネント2" bodies 2 removing the originals makes body 5 in component "上段"
copy_body "ボディ -> コンポーネント3" bodies 3 removing the originals makes body 6 in component "中段"
component "下段" placed x (1, 0, 0) y (0, 1, 0) z (0, 0, 1) at (0, 0, 0)
component "上段" placed x (1, 0, 0) y (0, 1, 0) z (0, 0, 1) at (0, 0, 0)
component "中段" placed x (1, 0, 0) y (0, 1, 0) z (0, 0, 1) at (0, 0, 0)
named bodies: "下段", "上段", "中段"

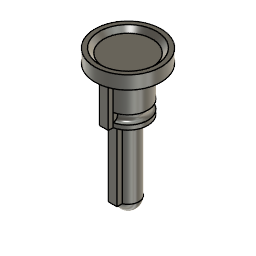
design "ボタンC"
Autodesk Fusion 360 part; units mm, degrees
sketch "スケッチ1" plane through (0, 0, 0) normal (0, 0, 1) x (1, 0, 0)
  circle A0 centre (0, 0) radius 7.5
  dimension "d1" = 15
  constraint coincident A0.centre origin
  measures "d1" diameter of A0
extrude "押し出し1" add sketch "スケッチ1" along normal blind 2
sketch "スケッチ2" plane through (0, 0, 2) normal (0, 0, 1) x (-1, 0, 0)
  circle A0 centre (0, 0) radius 7.5
  circle A1 centre (0, 0) radius 6.5
  dimension "d4" = 13
  constraint coincident A0.centre A1.centre
  measures "d4" diameter of A1
extrude "押し出し2" add sketch "スケッチ2" along normal blind 1
chamfer "面取り1" distance 1 angle 45 1 edges at (6.0601, 2.3505, 2)
sketch "スケッチ3" plane through (0, 0, 0) normal (0, 0, -1) x (1, 0, 0)
  circle A0 centre (0, 0) radius 7.5
  line L0 (0, -2.5) -> (0, 2.5)
  circle A1 centre (0, 0) radius 2.5
  line L1 (1, 1.5) -> (-1, 1.5)
  line L2 (-1, 1.5) -> (-1, 3.5)
  line L3 (-1, 3.5) -> (1, 3.5)
  line L4 (1, 3.5) -> (1, 1.5)
  line L5 (1, 1.5) -> (-1, 3.5) construction
  line L6 (-1, 1.5) -> (1, 3.5) construction
  circle A2 centre (0, 0) radius 4.5
  line L7 (0.9923, 5.5) -> (-1.0077, 5.5)
  line L8 (-1.0077, 5.5) -> (-1.0077, 3.5)
  line L9 (-1.0077, 3.5) -> (0.9923, 3.5)
  line L10 (0.9923, 3.5) -> (0.9923, 5.5)
  line L11 (0.9923, 5.5) -> (-1.0077, 3.5) construction
  line L12 (-1.0077, 5.5) -> (0.9923, 3.5) construction
  point P0 (0, 2.5)
  point P1 (0, 2.5)
  point P2 (-0.0077, 4.5)
  dimension "d8" = 5
  dimension "d15" = 2.5
  dimension "d22" = 2
  dimension "d23" = 2
  dimension "d24" = 9
  dimension "d25" = 2
  dimension "d26" = 2
  constraint coincident A0.centre A1.centre
  constraint midpoint L0 A0.centre
  constraint vertical L0
  constraint coincident P1 P0
  constraint horizontal L1
  constraint perpendicular L1 L2
  constraint parallel L1 L3
  constraint parallel L2 L4
  constraint coincident L5 P1
  constraint coincident L6 P1
  constraint horizontal L7
  constraint perpendicular L7 L8
  constraint parallel L7 L9
  constraint parallel L8 L10
  constraint coincident L11 P2
  constraint coincident L12 P2
  constraint coincident A2 P2
  measures "d8" diameter of A1
  measures "d15" distance of A0.centre P1
  measures "d22" distance of L2.end L3.end
  measures "d23" distance of L1.end L2.end
  measures "d24" diameter of A2
  measures "d25" distance of L7.end L8.end
  measures "d26" distance of L7.start L7.end
extrude "押し出し3" add sketch "スケッチ3" along normal blind 26 contours L0 A1 L1 L2 | L0 A1 L1 L4 | L0 A1 L1 L2 | L0 A1 L1 L4 | A1 L2 L3 L4 L9
sketch "スケッチ5" plane through (0, 0, 0) normal (0, 0, -1) x (1, 0, 0)
  line L0 (-1, 2.2913) -> (-1, 3.5)
  line L1 (-1, 3.5) -> (0.9923, 3.5)
  line L2 (1, 3.5) -> (1, 2.2913)
  arc A0 (-1, 2.2913) -> (1, 2.2913) centre (0, 0) ccw
  circle A1 centre (0, 0) radius 7.5
  line L3 (0.9923, 3.5) -> (1, 3.5)
extrude "押し出し4" add sketch "スケッチ3" along normal blind 10 contours A1 L2 L3 L4 A2 L8 L9 L10 | L3 A2 L8 L9 L10 | A2 L7 L8 L10
sphere "球プリミティブ1" add diameter 5 placed x (1, 0, 0) y (0, -1, 0) z (0, 0, -1) at (0, 0, -26)
ref_plane "作業平面1" through (0, 0, -8) normal (0, 0, 1) x (-1, 0, 0)
sketch "スケッチ7" plane through (0, 0, -8) normal (0, 0, 1) x (1, 0, 0)
  circle A0 centre (0, 0) radius 4.5
  arc A1 (0.9923, -4.3892) -> (-1.0077, -4.3857) centre (0, 0) ccw
  line L0 (0.9923, -4.3892) -> (0.9923, -5.5)
  line L1 (0.9923, -5.5) -> (-1.0077, -5.5)
  line L2 (-1.0077, -5.5) -> (-1.0077, -4.3857)
  line L3 (0.9923, -3.5) -> (1, -3.5)
  line L4 (1, -3.5) -> (1, -2.2913)
  arc A2 (1, -2.2913) -> (-1, -2.2913) centre (0, 0) ccw
  line L5 (-1, -2.2913) -> (-1, -3.5)
  line L6 (-1, -3.5) -> (0.9923, -3.5)
  line L7 (-1.0077, -5.5) -> (1, -5.5)
  line L8 (1, -5.5) -> (1, -3.5)
  line L9 (1, -3.5) -> (-1.0077, -3.5)
  line L10 (-1.0077, -3.5) -> (-1.0077, -5.5)
  line L11 (1, -2.2913) -> (-1, -2.2913)
  line L12 (-1, -2.2913) -> (-1, -3.5)
  line L13 (-1, -3.5) -> (1, -3.5)
  line L14 (1, -3.5) -> (1, -2.2913)
  dimension "d31" = 9
  constraint coincident A0.centre A1.centre
  constraint horizontal L7
  constraint vertical L8
  constraint horizontal L9
  constraint vertical L10
  constraint coincident L3.end L4.start
  constraint coincident L1.end L2.start
  constraint horizontal L11
  constraint vertical L12
  constraint horizontal L13
  constraint vertical L14
  constraint coincident L5.end L6.start
  constraint coincident L4.end A2.start
  measures "d31" diameter of A0
torus "トーラス プリミティブ1" cut centre line diameter 9 section diameter 2 placed x (1, 0, 0) y (0, 1, 0) z (0, 0, 1) at (0, 0, -8)
extrude "押し出し5" add sketch "スケッチ7" along normal blind 2 and the other way blind 1.9 contours A0 A1 L3 L6 L8 L9 L10 L13 | A0 L0 L1 L2 L7 L10 | L3 L4 L5 L6 L9 L11 L12 L13 L14
equation "d24 = d8 + 4 mm"

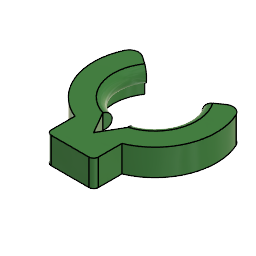
design "ボタンストッパー"
Autodesk Fusion 360 part; units mm, degrees
sketch "スケッチ1" plane through (0, 0, 0) normal (0, 0, 1) x (1, 0, 0)
  circle A0 centre (0, 0) radius 4.5
  line L0 (1, 5.5) -> (-1, 5.5)
  line L1 (-1, 5.5) -> (-1, 3.5)
  line L2 (-1, 3.5) -> (1, 3.5)
  line L3 (1, 3.5) -> (1, 5.5)
  line L4 (1, 5.5) -> (-1, 3.5) construction
  line L5 (-1, 5.5) -> (1, 3.5) construction
  line L6 (-4.5, 0) -> (4.5, 0)
  arc A1 (-5.324488, 3.728247) -> (-6.5, 0) centre (0, 0) ccw
  line L7 (-5.324488, 3.728247) -> (0, 0)
  arc A2 (-6.5, 0) -> (0, -6.5) centre (0, 0) ccw
  line L8 (0, 2.5) -> (0, 20)
  arc A3 (6.5, 0) -> (5.324488, 3.728247) centre (0, 0) ccw
  line L9 (5.324488, 3.728247) -> (0, 0)
  arc A4 (0, -6.5) -> (6.5, 0) centre (0, 0) ccw
  line L10 (-2.5, -6) -> (-2.5, -9)
  line L11 (-2.5, -9) -> (2.5, -9)
  line L12 (2.5, -9) -> (2.5, -6)
  line L13 (0, 9) -> (0, -9)
  line L14 (0, -6.5) -> (-1.258345, -4.320482)
  line L15 (0, -6.5) -> (1.258345, -4.320482)
  point P0 (0, 4.5)
  point P1 (0, -6.5)
  dimension "d1" = 9
  dimension "d2" = 2
  dimension "d3" = 2
  dimension "d5" = 35
  dimension "d6" = 2
  dimension "d9" = 5
  dimension "d17" = 9
  dimension "d18" = 2.5
  dimension "d19" = 90
  dimension "d20" = 30
  constraint coincident A0.centre A1.centre
  constraint horizontal L0
  constraint perpendicular L0 L1
  constraint parallel L0 L2
  constraint parallel L1 L3
  constraint coincident L4 P0
  constraint coincident L5 P0
  constraint coincident A0 P0
  constraint vertical A0.centre P0
  constraint midpoint L6 A0.centre
  constraint coincident A0 L6.end
  constraint horizontal L6
  constraint symmetric A1.end L8 A3.start
  constraint symmetric A1 L8 A3
  constraint symmetric A0.centre L8 A1.centre
  constraint symmetric P1 L8 A2.end
  constraint symmetric A2 L8 A4
  constraint parallel L10 L12
  constraint coincident P1 A2.end
  constraint coincident A4 L12.end
  constraint coincident A2 L10.start
  constraint equal L10 L12
  constraint midpoint L13 A0.centre
  constraint coincident L11 L13.end
  constraint perpendicular L11 L13
  constraint midpoint L11 L13.end
  constraint symmetric P1 L13 A2.end
  measures "d1" diameter of A0
  measures "d2" distance of L1.end L2.end
  measures "d3" distance of L0.end L1.end
  measures "d5" angle of L6 L7
  measures "d6" distance of A0 A1
  measures "d9" distance of L10.end L11.end
  measures "d17" distance of A0.centre L11
  measures "d18" distance of L11 P1
  measures "d19" angle of L6 L13
  measures "d20" angle of L13 L14
extrude "押し出し1" add sketch "スケッチ1" along normal blind 3 contours A0 A1 L7 A2 L14 | A2 L10 L11 L13 | A0 A3 L9 A4 L15 | A4 L11 L12 L13 picked at (-2.57109, -5.222027) picked at (-1.117638, -8.147933) picked at (2.57109, -5.222027) picked at (1.117638, -8.147933)
move_face "面をオフセット1" offset 0.1 4 faces at (4.496269, 0.183209, 1) (4.479554, -0.428478, 2) (-4.494886, -0.214483, 1) (-4.496269, 0.183209, 2)
ref_plane "作業平面1" through (0, -2.722325, 2) normal (0, 0, -1) x (-1, 0, 0)
sketch "スケッチ2" plane through (0, 0, 2) normal (0, 0, -1) x (-1, 0, 0)
  line L0 (2.5, -9) -> (-2.5, -9)
  line L1 (-2.5, -9) -> (-2.5, -6)
  arc A0 (2.5, -6) -> (5.324488, 3.728247) centre (0, 0) ccw
  arc A1 (-3.604269, 2.523736) -> (-1.331554, -4.193682) centre (0, 0) ccw
  arc A2 (1.331554, -4.193682) -> (3.604269, 2.523736) centre (0, 0) ccw
  line L2 (2.5, -6) -> (2.5, -9)
  arc A3 (-5.324488, 3.728247) -> (-2.5, -6) centre (0, 0) ccw
pipe "パイプ1" add diameter 2 path "スケッチ2" along A2
pipe "パイプ2" add diameter 2 path "スケッチ2" along A1
fillet "フィレット1" radius 1 2 edges at (-5.324488, 3.728247, 1.5) (5.324488, 3.728247, 1.5)
fillet "フィレット2" radius 0.5 2 edges at (2.5, -9, 1.5) (-2.5, -9, 1.5)
move_face "面をオフセット2" offset -0.2 2 faces at (-4.187326, 1.179042, 1.001243) (4.054853, 1.57544, 2.998757)

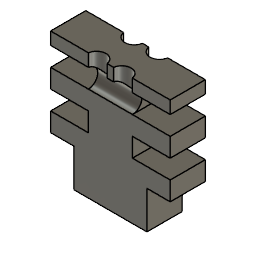
design "スイッチ-ワイヤー保持台"
Autodesk Fusion 360 part; units mm, degrees
sketch "スケッチ1" plane through (0, 0, 0) normal (0, 0, 1) x (1, 0, 0)
  line L0 (3, 1.5) -> (-3, 1.5)
  line L1 (-3, 1.5) -> (-3, -1.5)
  line L2 (-3, -1.5) -> (3, -1.5)
  line L3 (3, -1.5) -> (3, 1.5)
  line L4 (3, 1.5) -> (-3, -1.5) construction
  line L5 (-3, 1.5) -> (3, -1.5) construction
  dimension "d1" = 6
  dimension "d2" = 3
  constraint horizontal L0
  constraint perpendicular L0 L1
  constraint parallel L0 L2
  constraint parallel L1 L3
  constraint coincident L4 origin
  constraint coincident L5 origin
  measures "d1" distance of L1.end L2.end
  measures "d2" distance of L0.end L1.end
extrude "押し出し1" add sketch "スケッチ1" along normal blind 3
sketch "スケッチ2" plane through (0, 0, 3) normal (0, 0, 1) x (-1, 0, 0)
  line L0 (-3, 1.5) -> (-3, -1.5)
  line L1 (-3, -1.5) -> (3, -1.5)
  line L2 (3, -1.5) -> (3, 1.5)
  line L3 (3, 1.5) -> (-3, 1.5)
  line L4 (-4.75, -1.5) -> (4.75, -1.5)
  line L5 (4.75, -1.5) -> (4.75, 1.5)
  line L6 (4.75, 1.5) -> (-4.75, 1.5)
  line L7 (-4.75, 1.5) -> (-4.75, -1.5)
  line L8 (-4.75, -1.5) -> (4.75, 1.5) construction
  line L9 (4.75, -1.5) -> (-4.75, 1.5) construction
  dimension "d5" = 9.5
  dimension "d6" = 3
  constraint horizontal L4
  constraint perpendicular L4 L5
  constraint parallel L4 L6
  constraint parallel L5 L7
  constraint coincident L8 origin
  constraint coincident L9 origin
  measures "d5" distance of L5.end L6.end
  measures "d6" distance of L4.end L5.end
extrude "押し出し2" add sketch "スケッチ2" along normal blind 7
sketch "スケッチ3" plane through (0, 0, 10) normal (0, 0, 1) x (-1, 0, 0)
  line L0 (-4.75, 1.5) -> (-4.75, -1.5)
  line L1 (-4.75, -1.5) -> (4.75, -1.5)
  line L2 (4.75, -1.5) -> (4.75, 1.5)
  line L3 (4.75, 1.5) -> (-4.75, 1.5)
  line L4 (1, 0) -> (-1, 0)
  circle A0 centre (1, 0) radius 0.75 construction
  line L5 (1, 0) -> (2.5, 0)
  circle A1 centre (2.5, 0) radius 0.75 construction
  circle A2 centre (4, 0) radius 0.75 construction
  line L6 (2.5, 0) -> (4, 0)
  circle A3 centre (1, 1.5) radius 0.75
  dimension "d9" = 2
  dimension "d15" = 1.5
  dimension "d17" = 1.5
  dimension "d18" = 1.5
  dimension "d19" = 1.5
  dimension "d20" = 1.5
  dimension "d32" = 1.5
  dimension "d33" = 1
  constraint midpoint L4 origin
  constraint perpendicular L2 L4
  constraint coincident L4.start A0.centre
  constraint horizontal L5
  constraint coincident L5.end A1.centre
  constraint coincident A2.centre L6.end
  constraint perpendicular L2 L6
  constraint coincident L3 A3.centre
  measures "d9" distance of L4.start L4.end
  measures "d15" diameter of A0
  measures "d17" diameter of A1
  measures "d18" distance of L4.start L5.end
  measures "d19" diameter of A2
  measures "d20" distance of L5.end A2.centre
  measures "d32" diameter of A3
  measures "d33" horizontal distance of origin A3.centre
sketch "スケッチ5" plane through (0, -1.5, 0) normal (0, -1, 0) x (1, 0, 0)
  line L0 (-3, 0) -> (3, 0)
  line L1 (3, 0) -> (3, 3)
  line L2 (3, 3) -> (4.75, 3)
  line L3 (4.75, 3) -> (4.75, 10)
  line L4 (4.75, 10) -> (-4.75, 10)
  line L5 (-4.75, 10) -> (-4.75, 3)
  line L6 (-4.75, 3) -> (-3, 3)
  line L7 (-3, 3) -> (-3, 0)
  line L8 (-4.75, 3) -> (-4.75, 4.5)
  line L9 (-4.75, 4.5) -> (-1.75, 4.5)
  line L10 (-1.75, 4.5) -> (-1.75, 6)
  line L11 (-1.75, 6) -> (-4.75, 6)
  line L12 (-4.75, 6) -> (-4.75, 4.5)
  line L13 (-4.75, 6) -> (-4.75, 7.5)
  line L14 (-4.75, 7.5) -> (-1.75, 7.5)
  line L15 (-1.75, 7.5) -> (-1.75, 9)
  line L16 (-1.75, 9) -> (-4.75, 9)
  line L17 (-4.75, 9) -> (-4.75, 7.5)
  line L18 (0, 1.75) -> (0, 22.5)
  line L19 (4.75, 4.5) -> (1.75, 4.5)
  line L20 (1.75, 4.5) -> (1.75, 6)
  line L21 (1.75, 6) -> (4.75, 6)
  line L22 (1.75, 7.5) -> (1.75, 9)
  line L23 (1.75, 9) -> (4.75, 9)
  line L24 (4.75, 9) -> (4.75, 7.5)
  line L25 (4.75, 7.5) -> (1.75, 7.5)
  dimension "d21" = 1.5
  dimension "d22" = 1.5
  dimension "d23" = 1.5
  dimension "d24" = 1.5
  dimension "d25" = 3
  dimension "d26" = 3
  constraint coincident L5.end L6.start
  constraint perpendicular L4 L8
  constraint horizontal L9
  constraint vertical L10
  constraint horizontal L11
  constraint vertical L12
  constraint perpendicular L11 L13
  constraint horizontal L14
  constraint vertical L15
  constraint horizontal L16
  constraint vertical L17
  constraint symmetric L8.end L18 L19.start
  constraint symmetric L9.end L18 L19.end
  constraint symmetric L10.end L18 L20.end
  constraint symmetric L11.end L18 L21.end
  constraint symmetric L13.end L18 L24.end
  constraint symmetric L14.end L18 L22.start
  constraint symmetric L15.end L18 L22.end
  constraint symmetric L16.end L18 L23.end
  measures "d21" distance of L5.end L8.end
  measures "d22" distance of L8.end L11.end
  measures "d23" distance of L11.end L13.end
  measures "d24" distance of L13.end L16.end
  measures "d25" distance of L8.end L9.end
  measures "d26" distance of L13.end L14.end
extrude "押し出し3" cut sketch "スケッチ5" against normal through all contours L5 L9 L10 L11 L12 | L3 L19 L20 L21 | L5 L14 L15 L16 L17 | L3 L22 L23 L24 L25
move_face "面をオフセット1" offset -0.1 4 faces at (-3, 0.5, 1) (-1, 1.5, 2) (1, -1.5, 2) (3, -0.5, 1)
ref_plane "作業平面1" through (-1, 0, 0) normal (1, 0, 0) x (0, 1, 0)
sketch "スケッチ10" plane through (0, 0, 10) normal (0, 0, 1) x (-1, 0, 0)
  line L0 (-4.75, 1.4) -> (-4.75, -1.4)
  line L1 (-4.75, -1.4) -> (4.75, -1.4)
  line L2 (4.75, -1.4) -> (4.75, 1.4)
  line L3 (4.75, 1.4) -> (-4.75, 1.4)
  circle A0 centre (1, -1.5) radius 0.75
  circle A1 centre (1, 1.5) radius 0.75
  circle A2 centre (-1, 1.5) radius 0.75
  circle A3 centre (-1, -1.5) radius 0.75
  dimension "d48" = 1.5
  dimension "d49" = 1.5
  dimension "d61" = 1.5
  dimension "d62" = 1.5
  dimension "d63" = 2
  dimension "d64" = 3
  dimension "d66" = 1
  dimension "d67" = 1.5
  constraint horizontal A0.centre A3.centre
  constraint vertical A2.centre A3.centre
  constraint vertical A0.centre A1.centre
  constraint horizontal A1.centre A2.centre
  measures "d48" diameter of A0
  measures "d49" diameter of A1
  measures "d61" diameter of A2
  measures "d62" diameter of A3
  measures "d63" distance of A0.centre A3.centre
  measures "d64" distance of A2.centre A3.centre
  measures "d66" horizontal distance of origin A3.centre
  measures "d67" vertical distance of origin A3.centre
extrude "押し出し6" cut sketch "スケッチ10" against normal blind 1.75 contours L3 A2 | L3 A2 | L1 A3 | L1 A3 | L3 A1 | L3 A1 | L1 A0 | L1 A0
sketch "スケッチ12" plane through (0, 0, 0) normal (1, 0, 0) x (0, 1, 0)
  line L0 (1.4, 7.5) -> (1.4, 9)
  line L1 (1.4, 9) -> (-1.4, 9)
  line L2 (-1.4, 9) -> (-1.4, 7.5)
  line L3 (-1.4, 7.5) -> (1.4, 7.5)
  circle A0 centre (1.4, 8.25) radius 0.75
  line L4 (0, 2.5) -> (0, 20)
  circle A1 centre (-1.4, 8.25) radius 0.75
  dimension "d59" = 1.5
  constraint midpoint L0 A0.centre
  constraint symmetric A0 L4 A1
  measures "d59" diameter of A0
extrude "押し出し8" cut sketch "スケッチ12" along normal through all and the other way through all contours L0 A0 | L0 A0 | L2 A1 | L2 A1
equation "d5 = 7 mm + 1.25 * 2 mm"
equation "d12 = 0.1 mm"
equation "d25 = ( 1.5 * 2 ) * 1 mm"
equation "d26 = d25"
equation "d30 = 1 mm + d12 + d12"

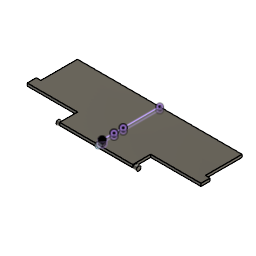
design "シーソー"
Autodesk Fusion 360 part; units mm, degrees